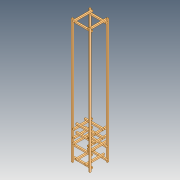
# Autodesk Inventor part: Base listones
Saved by Autodesk Inventor 2020 (Build 240168000, 168)
## iProperties
Created: 2022-05-04
Part Number: Base listones
Material: Generic
Document SubType Name: Modeling
Designer: leo
Density: 1 g/cm^3
Appearance: Yellow Pine - Solid Stained Light Low Gloss
Author: leo
Autodesk Inventor part; units mm, degrees
ref_plane "YZ Plane" through (0, 0, 0) normal (1, 0, 0) x (0, 1, 0)
ref_plane "XZ Plane" through (0, 0, 0) normal (0, 1, 0) x (-1, 0, 0)
ref_plane "XY Plane" through (0, 0, 0) normal (0, 0, 1) x (1, 0, 0)
sketch "Sketch1" plane through (0, 0, 0) normal (0, 1, 0) x (-1, 0, 0)
  line L0 (150, 150) -> (129, 150)
  line L1 (129, 150) -> (129, 129)
  line L2 (129, 129) -> (150, 129)
  line L3 (150, 129) -> (150, 150)
  line L4 (150, -150) -> (129, -150)
  line L5 (129, -150) -> (129, -129)
  line L6 (129, -129) -> (150, -129)
  line L7 (150, -129) -> (150, -150)
  line L8 (-150, -150) -> (-129, -150)
  line L9 (-129, -150) -> (-129, -129)
  line L10 (-129, -129) -> (-150, -129)
  line L11 (-150, -129) -> (-150, -150)
  line L12 (-150, 150) -> (-129, 150)
  line L13 (-129, 150) -> (-129, 129)
  line L14 (-129, 129) -> (-150, 129)
  line L15 (-150, 129) -> (-150, 150)
  line L16 (150, 129) -> (150, -129) construction
  line L17 (129, 150) -> (-129, 150) construction
  point P0 (0, 0)
  point P1 (150, 0)
  point P2 (0, 150)
  dimension "d0" = 21
  dimension "d1" = 300
  dimension "d2" = 300
  constraints: 36 end point, 8 parallel, 7 equal length, 5 horizontal, 4 perpendicular, 2 collinear, 2 midpoint, 2 point on line, 1 horizontal alignment, 1 vertical, 1 vertical alignment
  measures "d0" distance of L0.start L0.end
  measures "d1" distance between parallel lines of L15 L3
  measures "d2" distance between parallel lines of L4 L0
extrude "Extrusion1" add sketch "Sketch1" along normal blind 2000
sketch "Sketch2" plane through (0, 0, 0) normal (1, 0, 0) x (0, 1, 0)
  line L0 (60, 129) -> (38, 129)
  line L1 (38, 129) -> (38, 107)
  line L2 (38, 107) -> (60, 107)
  line L3 (60, 107) -> (60, 129)
  line L4 (60, -129) -> (38, -129)
  line L5 (38, -129) -> (38, -107)
  line L6 (38, -107) -> (60, -107)
  line L7 (60, -107) -> (60, -129)
  line L8 (49, 107) -> (49, -107) construction
  line L9 (240, 129) -> (218, 129)
  line L10 (218, 129) -> (218, 107)
  line L11 (218, 107) -> (240, 107)
  line L12 (240, 107) -> (240, 129)
  line L13 (240, -129) -> (218, -129)
  line L14 (218, -129) -> (218, -107)
  line L15 (218, -107) -> (240, -107)
  line L16 (240, -107) -> (240, -129)
  line L17 (1960, 107) -> (1960, 129)
  line L18 (1960, 129) -> (1938, 129)
  line L19 (1938, 107) -> (1960, 107)
  line L20 (1938, 129) -> (1938, 107)
  line L21 (1960, -107) -> (1960, -129)
  line L22 (1960, -129) -> (1938, -129)
  line L23 (1938, -129) -> (1938, -107)
  line L24 (1938, -107) -> (1960, -107)
  point P0 (0, 0)
  point P1 (49, 0)
  point P2 (229, 107)
  point P3 (229, -107)
  point P4 (1949, 107)
  point P5 (1949, -107)
  dimension "d5" = 258
  dimension "d6" = 60
  dimension "d7" = 22
  dimension "d19" = 180
  dimension "d46" = 1900
  constraints: 50 end point, 4 horizontal, 4 parallel, 3 equal length, 3 midpoint, 3 point on line, 2 collinear, 2 perpendicular, 1 horizontal alignment, 34 other
  measures "d5" distance between parallel lines of L4 L0
  measures "d6" distance from line of L3 point (0, 0)
  measures "d7" distance of L0.end L1.end
  measures "d19" distance of L0.start L9.start
  measures "d46" distance of L0.start L17.end
extrude "Extrusion2" add sketch "Sketch2" along normal mid plane 300 separate body contours L3 L2 L1 L0 | L4 L5 L6 L7 | L19 L20 L18 L17 | L21 L22 L23 L24
sketch "Sketch3" plane through (0, 0, 0) normal (0, 0, 1) x (1, 0, 0)
  line L0 (-85, 82) -> (-63, 82)
  line L1 (-63, 82) -> (-63, 60)
  line L2 (-63, 60) -> (-85, 60)
  line L3 (-85, 60) -> (-85, 82)
  line L4 (0, 0) -> (0, 206.2216) construction
  line L5 (85, 82) -> (63, 82)
  line L6 (63, 82) -> (63, 60)
  line L7 (63, 60) -> (85, 60)
  line L8 (85, 60) -> (85, 82)
  line L9 (-129, 282) -> (-107, 282)
  line L10 (-107, 282) -> (-107, 260)
  line L11 (-107, 260) -> (-129, 260)
  line L12 (-129, 260) -> (-129, 282)
  line L13 (129, 282) -> (107, 282)
  line L14 (107, 282) -> (107, 260)
  line L15 (107, 260) -> (129, 260)
  line L16 (129, 260) -> (129, 282)
  line L17 (107, 1982) -> (107, 1960)
  line L18 (129, 1982) -> (107, 1982)
  line L19 (129, 1960) -> (129, 1982)
  line L20 (107, 1960) -> (129, 1960)
  line L21 (-107, 1982) -> (-107, 1960)
  line L22 (-129, 1982) -> (-107, 1982)
  line L23 (-129, 1960) -> (-129, 1982)
  line L24 (-107, 1960) -> (-129, 1960)
  dimension "d10" = 60
  dimension "d11" = 22
  dimension "d12" = 170
  dimension "d15" = 258
  dimension "d16" = 200
  dimension "d53" = 1700
  constraints: 50 end point, 8 symmetric about line, 4 parallel, 3 equal length, 2 horizontal, 2 perpendicular, 2 vertical, 1 collinear, 15 other
  measures "d10" distance from line of L2 L4.start
  measures "d11" distance of L0.start L0.end
  measures "d12" distance between parallel lines of L8 L3
  measures "d15" distance between parallel lines of L16 L12
  measures "d16" distance between parallel lines of L9 L0
  measures "d53" distance of L13.end L17.start
extrude "Extrusion3" add sketch "Sketch3" along normal mid plane 300 separate body contours L0 L1 L2 L3 | L8 L7 L6 L5 | L18 L19 L20 L17 | L21 L24 L23 L22
extrude "Extrusion4" add sketch "Sketch2" along normal mid plane 300 separate body contours L12 L11 L10 L9 | L13 L14 L15 L16
extrude "Extrusion5" add sketch "Sketch3" along normal mid plane 300 separate body contours L9 L10 L11 L12 | L16 L15 L14 L13
sketch "Sketch4" plane through (0, 0, 0) normal (0, 0, 1) x (1, 0, 0)
  line L0 (128, 480) -> (106, 480)
  line L1 (106, 480) -> (106, 458)
  line L2 (106, 458) -> (128, 458)
  line L3 (128, 458) -> (128, 480)
  line L4 (0, 0) -> (0, 747.9187)
  line L5 (-128, 480) -> (-106, 480)
  line L6 (-106, 480) -> (-106, 458)
  line L7 (-106, 458) -> (-128, 458)
  line L8 (-128, 458) -> (-128, 480)
  dimension "d31" = 256
  dimension "d32" = 22
  dimension "d33" = 480
  constraints: 18 end point, 4 symmetric about line, 2 parallel, 2 perpendicular, 1 horizontal, 1 vertical
  measures "d31" distance between parallel lines of L8 L3
  measures "d32" distance of L1.end L2.end
  measures "d33" distance from line of L4.start L0
extrude "Extrusion6" add sketch "Sketch4" along normal mid plane 300 separate body
sketch "Sketch5" plane through (0, 0, 0) normal (1, 0, 0) x (0, 1, 0)
  line L0 (502, 79.5) -> (480, 79.5)
  line L1 (480, 79.5) -> (480, 57.5)
  line L2 (480, 57.5) -> (502, 57.5)
  line L3 (502, 57.5) -> (502, 79.5)
  line L4 (0, 0) -> (506.9867, 0)
  line L5 (502, -79.5) -> (480, -79.5)
  line L6 (480, -79.5) -> (480, -57.5)
  line L7 (480, -57.5) -> (502, -57.5)
  line L8 (502, -57.5) -> (502, -79.5)
  dimension "d36" = 480
  dimension "d37" = 22
  dimension "d38" = 115
  constraints: 18 end point, 4 symmetric about line, 2 horizontal, 2 parallel, 2 perpendicular
  measures "d36" distance from line of L4.start L1
  measures "d37" distance of L2.end L0.start
  measures "d38" distance between parallel lines of L7 L2
extrude "Extrusion7" add sketch "Sketch5" along normal mid plane 300 separate body
pattern_linear "Rectangular Pattern2" count 2 spacing 120 along (0, -1, 0) of "Extrusion7", "Extrusion6" bodies 7
equation "\"d2\" = d1"
body "Solid1"
body "Solid2"
body "Solid3"
body "Solid4"
body "Solid5"
body "Solid8"
body "Solid9"
